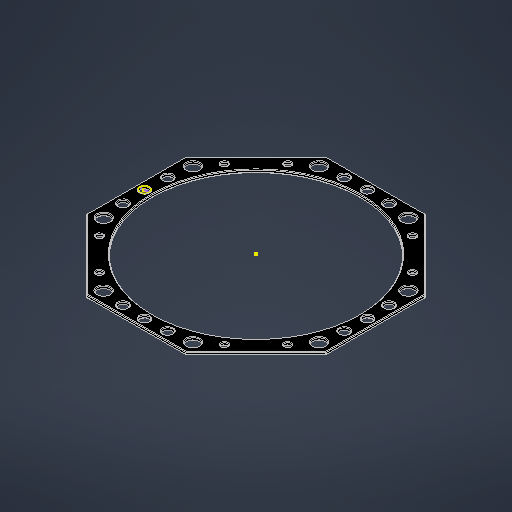
# Autodesk Inventor part: Part5
Saved by Autodesk Inventor 2026.2 (Build 302298000, 298)
## iProperties
Created: 2025-12-08
Part Number: Part5
Material: Generic
Document SubType Name: Modeling
Designer: Thoma
Density: 1 g/cm^3
Appearance: Anodized - Black
Author: Thoma
Autodesk Inventor part; units mm, degrees
ref_plane "YZ Plane" through (0, 0, 0) normal (1, 0, 0) x (0, 1, 0)
ref_plane "XZ Plane" through (0, 0, 0) normal (0, 1, 0) x (-1, 0, 0)
ref_plane "XY Plane" through (0, 0, 0) normal (0, 0, 1) x (1, 0, 0)
sketch "Sketch1" plane through (0, 0, 0) normal (0, 1, 0) x (-1, 0, 0)
  line L0 (-78.7006, -190) -> (-190, -78.7006)
  line L1 (-190, -78.7006) -> (-190, 78.7006)
  line L2 (-190, 78.7006) -> (-78.7006, 190)
  line L3 (-78.7006, 190) -> (78.7006, 190)
  line L4 (78.7006, 190) -> (190, 78.7006)
  line L5 (190, 78.7006) -> (190, -78.7006)
  line L6 (190, -78.7006) -> (78.7006, -190)
  line L7 (78.7006, -190) -> (-78.7006, -190)
  circle A0 centre (0, 0) radius 165
  point P0 (0, 190)
  point P1 (0, -190)
  dimension "d0" = 380
  dimension "d1" = 330
  constraints: 16 end point, 2 coincident, 2 midpoint, 1 centre point, 17 other
  measures "d0" distance of point (0, 190) point (0, -190)
  measures "d1" diameter of A0
extrude "Extrusion1" add sketch "Sketch1" along normal blind 5
fillet "Fillet1" radius 1 20 edges at (-134.3503, 5, -134.3503) (-190, 5, 0) (-134.3503, 5, 134.3503) (0, 5, 190) (134.3503, 5, 134.3503) (190, 5, 0) (134.3503, 5, -134.3503) (0, 5, -190) (190, 0, 0) (190, 2.5, -78.7006) (190, 2.5, 78.7006) (-134.3503, 0, -134.3503) (0, 0, -190) (134.3503, 0, -134.3503) (134.3503, 0, 134.3503) (0, 0, 190) (-134.3503, 0, 134.3503) (-190, 0, 0) (165, 5, 0) (165, 0, 0)
sketch "Sketch3" plane through (0, 0, 0) normal (0, -1, 0) x (1, 0, 0)
  line L0 (189, 78.2864) -> (78.2864, 189) projected
  circle A0 centre (0, 0) radius 165 projected
  line L1 (189, -78.2864) -> (189, 78.2864) projected
  line L2 (78.2864, -189) -> (189, -78.2864) projected
  circle A1 centre (0, 0) radius 166 projected
  circle A2 centre (171.182, -70.9059) radius 10
  line L3 (189, -78.2864) -> (180.4208, -74.7327)
  line L4 (161.9432, -67.0791) -> (153.364, -63.5254)
  dimension "d57" = 20
  constraints: 4 end point, 2 point on circle, 1 centre point, 4 other
  measures "d57" diameter of A2
extrude "Extrusion2" cut sketch "Sketch3" against normal blind 5 contours A2
pattern_circular "Circular Pattern1" count 8 over 360 about axis through (0, -10, 0) along (0, 1, 0) of "Extrusion2"
fillet "Fillet4" radius 1 2 edges at (-63.8348, 0, 164.1109) (-63.8348, 5, 164.1109)
pattern_circular "Circular Pattern6" count 8 over 360 about axis through (0, -10, 0) along (0, 1, 0) of "Fillet4"
sketch "Sketch5" plane through (0, 5, 0) normal (0, 1, 0) x (1, 0, 0)
  line L0 (190, -78.2864) -> (189, -78.2864) projected
  line L1 (189, -78.2864) -> (153.364, -63.5254)
  circle A0 centre (0, 0) radius 166 projected
  line L2 (189, 78.2864) -> (153.364, 63.5254)
  circle A1 centre (171.182, 70.9059) radius 10
  line L3 (177.3155, 0) -> (166, 0)
  line L4 (187, 0) -> (166, 0)
  line L5 (166, 0) -> (189, 0)
  arc A2 (171.182, -70.9059) -> (177.3155, 0) centre (-235.6051, 0) ccw
  circle A3 centre (177.3155, 0) radius 7.5
  arc A4 (177.3155, 0) -> (171.182, 70.9059) centre (-235.6051, 0) ccw
  circle A5 centre (175.7792, 35.5853) radius 7.5
  circle A6 centre (175.7792, -35.5853) radius 7.5
  circle A7 centre (35.5853, 175.7792) radius 7.5
  circle A8 centre (0, 177.3155) radius 7.5
  circle A9 centre (-35.5853, 175.7792) radius 7.5
  circle A10 centre (-175.7792, 35.5853) radius 7.5
  circle A11 centre (-177.3155, 0) radius 7.5
  circle A12 centre (-175.7792, -35.5853) radius 7.5
  circle A13 centre (-35.5853, -175.7792) radius 7.5
  circle A14 centre (0, -177.3155) radius 7.5
  circle A15 centre (35.5853, -175.7792) radius 7.5
  point P0 (162.508, 31.7784)
  dimension "d22" = 45
  dimension "d62" = 20
  dimension "d63" = 15
  dimension "d64" = 15
  dimension "d65" = 15
  dimension "d68" = 360
  constraints: 15 centre point, 10 end point, 10 point on circle, 2 coincident, 2 midpoint, 2 point on line, 1 horizontal, 1 line through centre, 29 other
  measures "d62" diameter of A1
  measures "d63" diameter of A3
  measures "d64" diameter of A5
  measures "d65" diameter of A6
extrude "Extrusion3" cut sketch "Sketch5" against normal blind 5 contours A6 A2 | A2 A6 | A3 A4 L3 | L3 A2 A3 | A2 L4 A3 | A4 A3 L4 | A5 A4 | A4 A5
pattern_circular "Circular Pattern7" count 4 over 360 about axis through (0, -10, 0) along (0, 1, 0) of "Extrusion3"
sketch "Sketch8" plane through (0, 5, 0) normal (0, 1, 0) x (1, 0, 0)
  line L0 (189, 78.2864) -> (189, -78.2864) projected
  line L1 (189, -78.2864) -> (153.364, -63.5254)
  circle A0 centre (0, 0) radius 166 projected
  line L2 (78.2864, -189) -> (63.5254, -153.364)
  line L3 (189, 0) -> (166, 0)
  line L4 (133.6432, -133.6432) -> (117.3797, -117.3797)
  arc A1 (70.9059, -171.182) -> (125.5115, -125.5115) centre (-158.068, 158.068) ccw
  arc A2 (125.5115, -125.5115) -> (171.182, -70.9059) centre (-158.068, 158.068) ccw
  circle A3 centre (149.5607, -99.224) radius 5
  circle A4 centre (99.224, -149.5607) radius 5
  dimension "d75" = 45
  dimension "d79" = 45
  dimension "d81" = 10
  dimension "d82" = 10
  constraints: 8 end point, 8 point on circle, 4 centre point, 4 midpoint, 1 horizontal, 1 line through centre, 8 other
  measures "d81" diameter of A3
  measures "d82" diameter of A4
extrude "Extrusion5" cut sketch "Sketch8" against normal blind 5 contours A3 A2 | A2 A3 | A4 A1 | A1 A4
pattern_circular "Circular Pattern8" count 4 over 360 about axis through (0, -10, 0) along (0, 1, 0) of "Extrusion5"
fillet "Fillet5" radius 1 10 edges at (35.5853, 5, 168.2792) (35.5853, 0, 168.2792) (0, 5, 169.8155) (0, 0, 169.8155) (-35.5853, 5, 168.2792) (-35.5853, 0, 168.2792) (94.224, 5, 149.5607) (94.224, 0, 149.5607) (144.5607, 5, 99.224) (144.5607, 0, 99.224)
pattern_circular "Circular Pattern9" count 4 over 360 about axis through (0, -10, 0) along (0, 1, 0) of "Fillet5"
sketch "Sketch9" plane through (0, 5, 0) normal (0, 1, 0) x (1, 0, 0)
  line L0 (-184.8155, 0) -> (-169.8155, 0)
  circle A0 centre (-177.3155, 0) radius 7.5 projected
  point P0 (0, 0)
  constraints: 2 end point, 2 point on circle, 1 horizontal
body "Solid1"
